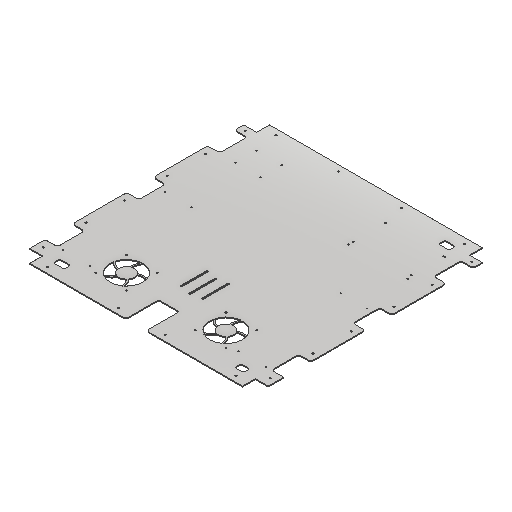
# Autodesk Inventor part: LC_ALU_2mm_Bottom_Plate
Saved by Autodesk Inventor 2026.1 (Build 301233000, 233)
## iProperties
Created: 2016-06-21
Part Number: LC_ALU_2mm_Bottom_Plate
Material: Ogólny
Document SubType Name: Modeling
Designer: Andrzej
Density: 1 g/cm^3
Appearance: Obrobione - aluminium
Mass: 583.865 g
Surface Area: 5900.9 cm^2
Volume: 583.865 cm^3
Author: Andrzej
Autodesk Inventor part; units mm, degrees
ref_plane "YZ Plane" through (0, 0, 0) normal (1, 0, 0) x (0, 1, 0)
ref_plane "XZ Plane" through (0, 0, 0) normal (0, 1, 0) x (-1, 0, 0)
ref_plane "XY Plane" through (0, 0, 0) normal (0, 0, 1) x (1, 0, 0)
sketch "Szkic1" plane through (0, 0, 0) normal (0, 0, 1) x (1, 0, 0)
  line L0 (-788.9548, 119.5598) -> (-788.9548, 95.5598)
  line L1 (-788.9548, 95.5598) -> (-760.4548, 95.5598)
  line L2 (-760.4548, 35.1598) -> (-788.9548, 35.1598)
  line L3 (-788.9548, 35.1598) -> (-788.9548, -94.1902)
  line L4 (-788.9548, -94.1902) -> (-760.4548, -94.1902)
  line L5 (-760.4548, -153.6902) -> (-788.9548, -153.6902)
  line L6 (-788.9548, -153.6902) -> (-788.9548, -283.0402)
  line L7 (-788.9548, -283.0402) -> (-760.4548, -283.0402)
  line L8 (-760.4548, -343.4402) -> (-788.9548, -343.4402)
  line L9 (-788.9548, -343.4402) -> (-788.9548, -382.4402)
  line L10 (-788.9548, -382.4402) -> (-758.9548, -382.4402)
  line L11 (-758.9548, -382.4402) -> (-758.9548, -412.4402)
  line L12 (-758.9548, -412.4402) -> (-259.9548, -412.4402)
  line L13 (-788.9548, 119.5598) -> (-758.9548, 119.5598)
  line L14 (-758.9548, 119.5598) -> (-758.9548, 149.5598)
  line L15 (-758.9548, 149.5598) -> (-259.9548, 149.5598)
  line L16 (-259.9548, -412.4402) -> (-259.9548, -382.4402)
  line L17 (-259.9548, -382.4402) -> (-229.9548, -382.4402)
  line L18 (-259.9548, 149.5598) -> (-259.9548, 119.5598)
  line L19 (-259.9548, 119.5598) -> (-229.9548, 119.5598)
  line L20 (-229.9548, 119.5598) -> (-229.9548, 95.5598)
  line L21 (-229.9548, 95.5598) -> (-258.4548, 95.5598)
  line L22 (-258.4548, 95.5598) -> (-258.4548, 35.1598)
  line L23 (-258.4548, 35.1598) -> (-229.9548, 35.1598)
  line L24 (-229.9548, 35.1598) -> (-229.9548, -94.1902)
  line L25 (-229.9548, -94.1902) -> (-258.4548, -94.1902)
  line L26 (-258.4548, -94.1902) -> (-258.4548, -153.6902)
  line L27 (-258.4548, -153.6902) -> (-229.9548, -153.6902)
  line L28 (-229.9548, -153.6902) -> (-229.9548, -283.0402)
  line L29 (-229.9548, -283.0402) -> (-258.4548, -283.0402)
  line L30 (-258.4548, -343.4402) -> (-229.9548, -343.4402)
  line L31 (-229.9548, -343.4402) -> (-229.9548, -382.4402)
  line L32 (-760.4548, 95.5598) -> (-760.4548, 35.1598)
  line L33 (-760.4548, -283.0402) -> (-760.4548, -343.4402)
  line L34 (-258.4548, -283.0402) -> (-258.4548, -343.4402)
  line L35 (-760.4548, -94.1902) -> (-760.4548, -153.6902)
  line L36 (-261.4548, 148.0598) -> (-757.4548, 148.0598)
  line L37 (-757.4548, 148.0598) -> (-757.4548, 118.0598)
  line L38 (-757.4548, 118.0598) -> (-787.4548, 118.0598)
  line L39 (-787.4548, 118.0598) -> (-787.4548, 97.0598)
  line L40 (-787.4548, 97.0598) -> (-758.9548, 97.0598)
  line L41 (-758.9548, 97.0598) -> (-758.9548, 33.6598)
  line L42 (-758.9548, 33.6598) -> (-787.4548, 33.6598)
  line L43 (-787.4548, 33.6598) -> (-787.4548, -92.6902)
  line L44 (-787.4548, -92.6902) -> (-758.9548, -92.6902)
  line L45 (-758.9548, -92.6902) -> (-758.9548, -155.1902)
  line L46 (-758.9548, -155.1902) -> (-787.4548, -155.1902)
  line L47 (-787.4548, -155.1902) -> (-787.4548, -281.5402)
  line L48 (-787.4548, -281.5402) -> (-758.9548, -281.5402)
  line L49 (-758.9548, -281.5402) -> (-758.9548, -344.9402)
  line L50 (-758.9548, -344.9402) -> (-787.4548, -344.9402)
  line L51 (-787.4548, -344.9402) -> (-787.4548, -380.9402)
  line L52 (-787.4548, -380.9402) -> (-757.4548, -380.9402)
  line L53 (-757.4548, -380.9402) -> (-757.4548, -410.9402)
  line L54 (-757.4548, -410.9402) -> (-261.4548, -410.9402)
  line L55 (-261.4548, -410.9402) -> (-261.4548, -380.9402)
  line L56 (-261.4548, -380.9402) -> (-231.4548, -380.9402)
  line L57 (-231.4548, -380.9402) -> (-231.4548, -344.9402)
  line L58 (-231.4548, -344.9402) -> (-259.9548, -344.9402)
  line L59 (-259.9548, -344.9402) -> (-259.9548, -281.5402)
  line L60 (-259.9548, -281.5402) -> (-231.4548, -281.5402)
  line L61 (-231.4548, -281.5402) -> (-231.4548, -155.1902)
  line L62 (-231.4548, -155.1902) -> (-259.9548, -155.1902)
  line L63 (-259.9548, -155.1902) -> (-259.9548, -92.6902)
  line L64 (-259.9548, -92.6902) -> (-231.4548, -92.6902)
  line L65 (-231.4548, -92.6902) -> (-231.4548, 33.6598)
  line L66 (-231.4548, 33.6598) -> (-259.9548, 33.6598)
  line L67 (-259.9548, 33.6598) -> (-259.9548, 97.0598)
  line L68 (-259.9548, 97.0598) -> (-231.4548, 97.0598)
  line L69 (-231.4548, 97.0598) -> (-231.4548, 118.0598)
  line L70 (-231.4548, 118.0598) -> (-261.4548, 118.0598)
  line L71 (-261.4548, 118.0598) -> (-261.4548, 148.0598)
  line L72 (-533.4548, -410.9402) -> (-533.4548, -334.4402)
  line L73 (-533.4548, -334.4402) -> (-485.4548, -334.4402)
  line L74 (-485.4548, -334.4402) -> (-485.4548, -410.9402)
  line L75 (-534.4548, -280.4402) -> (-534.4548, -220.4402) construction
  line L76 (-532.4548, -280.4402) -> (-532.4548, -220.4402)
  line L77 (-536.4548, -220.4402) -> (-536.4548, -280.4402)
  arc A0 (-536.4548, -280.4402) -> (-532.4548, -280.4402) centre (-534.4548, -280.4402) ccw
  arc A1 (-532.4548, -220.4402) -> (-536.4548, -220.4402) centre (-534.4548, -220.4402) ccw
  line L78 (-509.4548, -285.4402) -> (-509.4548, -225.4402) construction
  line L79 (-507.4548, -285.4402) -> (-507.4548, -225.4402)
  line L80 (-511.4548, -225.4402) -> (-511.4548, -285.4402)
  arc A2 (-511.4548, -285.4402) -> (-507.4548, -285.4402) centre (-509.4548, -285.4402) ccw
  arc A3 (-507.4548, -225.4402) -> (-511.4548, -225.4402) centre (-509.4548, -225.4402) ccw
  line L81 (-484.4548, -280.4402) -> (-484.4548, -220.4402) construction
  line L82 (-482.4548, -280.4402) -> (-482.4548, -220.4402)
  line L83 (-486.4548, -220.4402) -> (-486.4548, -280.4402)
  arc A4 (-486.4548, -280.4402) -> (-482.4548, -280.4402) centre (-484.4548, -280.4402) ccw
  arc A5 (-482.4548, -220.4402) -> (-486.4548, -220.4402) centre (-484.4548, -220.4402) ccw
  line L84 (-726.9548, -382.4402) -> (-709.9548, -382.4402)
  line L85 (-705.9548, -378.4402) -> (-705.9548, -371.4402)
  line L86 (-709.9548, -367.4402) -> (-726.9548, -367.4402)
  line L87 (-730.9548, -371.4402) -> (-730.9548, -378.4402)
  arc A6 (-705.9548, -371.4402) -> (-709.9548, -367.4402) centre (-709.9548, -371.4402) ccw
  arc A7 (-726.9548, -367.4402) -> (-730.9548, -371.4402) centre (-726.9548, -371.4402) ccw
  arc A8 (-730.9548, -378.4402) -> (-726.9548, -382.4402) centre (-726.9548, -378.4402) ccw
  arc A9 (-709.9548, -382.4402) -> (-705.9548, -378.4402) centre (-709.9548, -378.4402) ccw
  line L88 (-315.9548, 104.5598) -> (-298.9548, 104.5598)
  line L89 (-294.9548, 108.5598) -> (-294.9548, 115.5598)
  line L90 (-298.9548, 119.5598) -> (-315.9548, 119.5598)
  line L91 (-319.9548, 115.5598) -> (-319.9548, 108.5598)
  arc A10 (-315.9548, 119.5598) -> (-319.9548, 115.5598) centre (-315.9548, 115.5598) ccw
  arc A11 (-319.9548, 108.5598) -> (-315.9548, 104.5598) centre (-315.9548, 108.5598) ccw
  arc A12 (-298.9548, 104.5598) -> (-294.9548, 108.5598) centre (-298.9548, 108.5598) ccw
  arc A13 (-294.9548, 115.5598) -> (-298.9548, 119.5598) centre (-298.9548, 115.5598) ccw
  line L92 (-665.4548, -357.4402) -> (-585.4548, -357.4402)
  line L93 (-585.4548, -357.4402) -> (-585.4548, -277.4402)
  line L94 (-585.4548, -277.4402) -> (-665.4548, -277.4402)
  line L95 (-665.4548, -277.4402) -> (-665.4548, -357.4402)
  circle A14 centre (-625.4548, -317.4402) radius 38
  line L96 (-752.9548, -352.4402) -> (-675.4548, -352.4402)
  line L97 (-675.4548, -352.4402) -> (-675.4548, -70.9402)
  line L98 (-675.4548, -70.9402) -> (-752.9548, -70.9402)
  line L99 (-752.9548, -70.9402) -> (-752.9548, -352.4402)
  line L100 (-343.4548, -352.4402) -> (-265.9548, -352.4402)
  line L101 (-265.9548, -352.4402) -> (-265.9548, -70.9402)
  line L102 (-265.9548, -70.9402) -> (-343.4548, -70.9402)
  line L103 (-343.4548, -70.9402) -> (-343.4548, -352.4402)
  line L104 (-427.9548, 89.5598) -> (-284.9548, 89.5598)
  line L105 (-427.9548, 89.5598) -> (-427.9548, 5.5598)
  line L106 (-427.9548, 5.5598) -> (-284.9548, 5.5598)
  line L107 (-284.9548, 5.5598) -> (-284.9548, 89.5598)
  line L108 (-427.9548, 5.5598) -> (-427.9548, -5.4402)
  line L109 (-427.9548, -5.4402) -> (-281.4548, -5.4402)
  line L110 (-281.4548, -5.4402) -> (-281.4548, 89.5598)
  line L111 (-281.4548, 89.5598) -> (-284.9548, 89.5598)
  line L112 (-723.9548, 84.5598) -> (-638.9548, 84.5598)
  line L113 (-638.9548, 84.5598) -> (-638.9548, 28.5598)
  line L114 (-638.9548, 28.5598) -> (-723.9548, 28.5598)
  line L115 (-723.9548, 28.5598) -> (-723.9548, 84.5598)
  line L116 (-288.9548, 85.5598) -> (-285.4548, 85.5598) construction
  line L117 (-288.9548, 83.5598) -> (-285.4548, 83.5598)
  line L118 (-285.4548, 87.5598) -> (-288.9548, 87.5598)
  arc A15 (-288.9548, 87.5598) -> (-288.9548, 83.5598) centre (-288.9548, 85.5598) ccw
  arc A16 (-285.4548, 83.5598) -> (-285.4548, 87.5598) centre (-285.4548, 85.5598) ccw
  line L119 (-303.9548, -382.4402) -> (-291.9548, -382.4402)
  line L120 (-287.9548, -378.4402) -> (-287.9548, -371.4402)
  line L121 (-291.9548, -367.4402) -> (-303.9548, -367.4402)
  line L122 (-307.9548, -371.4402) -> (-307.9548, -378.4402)
  arc A17 (-287.9548, -371.4402) -> (-291.9548, -367.4402) centre (-291.9548, -371.4402) ccw
  arc A18 (-303.9548, -367.4402) -> (-307.9548, -371.4402) centre (-303.9548, -371.4402) ccw
  arc A19 (-307.9548, -378.4402) -> (-303.9548, -382.4402) centre (-303.9548, -378.4402) ccw
  arc A20 (-291.9548, -382.4402) -> (-287.9548, -378.4402) centre (-291.9548, -378.4402) ccw
  circle A21 centre (-625.4548, -317.4402) radius 18
  arc A22 (-662.7676, -310.2462) -> (-642.9339, -321.7394) centre (-636.2541, -287.3519) ccw
  arc A23 (-661.9161, -306.7362) -> (-643.4412, -318.141) centre (-635.1638, -284.0659) ccw
  arc A24 (-628.347, -279.5504) -> (-634.0544, -301.6274) centre (-598.7848, -298.9692) ccw
  arc A25 (-624.5951, -279.4499) -> (-630.4705, -300.1532) centre (-595.2035, -298.9764) ccw
  arc A26 (-589.7746, -304.3664) -> (-611.5366, -306.0261) centre (-598.1132, -338.5314) ccw
  arc A27 (-588.6863, -307.8446) -> (-609.4805, -309.1443) centre (-596.9934, -341.9338) ccw
  arc A28 (-601.3141, -346.7869) -> (-610.4589, -327.3963) centre (-635.7941, -351.1964) ccw
  arc A29 (-604.0661, -348.8492) -> (-612.6245, -330.0649) centre (-638.5893, -353.2367) ccw
  arc A30 (-644.1658, -350.5144) -> (-628.3669, -335.2031) centre (-659.1539, -319.2423) ccw
  arc A31 (-647.0681, -348.6951) -> (-631.6229, -334.3504) centre (-661.9, -317.2379) ccw
  line L123 (-433.4548, -357.4402) -> (-353.4548, -357.4402)
  line L124 (-353.4548, -357.4402) -> (-353.4548, -277.4402)
  line L125 (-353.4548, -277.4402) -> (-433.4548, -277.4402)
  line L126 (-433.4548, -277.4402) -> (-433.4548, -357.4402)
  circle A32 centre (-393.4548, -317.4402) radius 38
  circle A33 centre (-393.4548, -317.4402) radius 18
  arc A34 (-430.7676, -310.2462) -> (-410.9339, -321.7394) centre (-404.2541, -287.3519) ccw
  arc A35 (-429.9161, -306.7362) -> (-411.4412, -318.141) centre (-403.1638, -284.0659) ccw
  arc A36 (-396.347, -279.5504) -> (-402.0544, -301.6274) centre (-366.7848, -298.9692) ccw
  arc A37 (-392.5951, -279.4499) -> (-398.4705, -300.1532) centre (-363.2035, -298.9764) ccw
  arc A38 (-357.7746, -304.3664) -> (-379.5366, -306.0261) centre (-366.1132, -338.5314) ccw
  arc A39 (-356.6863, -307.8446) -> (-377.4805, -309.1443) centre (-364.9934, -341.9338) ccw
  arc A40 (-369.3141, -346.7869) -> (-378.4589, -327.3963) centre (-403.7941, -351.1964) ccw
  arc A41 (-372.0661, -348.8492) -> (-380.6245, -330.0649) centre (-406.5893, -353.2367) ccw
  arc A42 (-412.1658, -350.5144) -> (-396.3669, -335.2031) centre (-427.1539, -319.2423) ccw
  arc A43 (-415.0681, -348.6951) -> (-399.6229, -334.3504) centre (-429.9, -317.2379) ccw
  point P0 (0, 0)
  point P1 (-534.4548, -250.4402)
  point P2 (-484.4548, -250.4402)
  point P3 (-509.4548, -255.4402)
  point P4 (-730.9548, -382.4402)
  point P5 (-705.9548, -367.4402)
  point P6 (-705.9548, -382.4402)
  point P7 (-730.9548, -367.4402)
  point P8 (-319.9548, 104.5598)
  point P9 (-294.9548, 119.5598)
  point P10 (-294.9548, 104.5598)
  point P11 (-319.9548, 119.5598)
  point P12 (-661.2048, -353.1902)
  point P13 (-589.7048, -353.1902)
  point P14 (-589.7048, -281.6902)
  point P15 (-661.2048, -281.6902)
  point P16 (-745.9548, -345.4402)
  point P17 (-743.4548, -108.9402)
  point P18 (-682.4548, -345.4402)
  point P19 (-682.4548, -108.9402)
  point P20 (-336.4548, -345.4402)
  point P21 (-333.9548, -108.9402)
  point P22 (-272.9548, -345.4402)
  point P23 (-272.9548, -108.9402)
  point P24 (-369.5, 3)
  point P25 (-423.9548, 85.5598)
  point P26 (-423.9548, 9.5598)
  point P27 (-288.9548, 9.5598)
  point P28 (-423.9548, -1.4402)
  point P29 (-285.4548, -1.4402)
  point P30 (-720.4548, 81.0598)
  point P31 (-720.4548, 32.0598)
  point P32 (-662.4548, 32.0598)
  point P33 (-662.4548, 81.0598)
  point P34 (-287.2048, 85.5598)
  point P35 (-307.9548, -382.4402)
  point P36 (-287.9548, -367.4402)
  point P37 (-287.9548, -382.4402)
  point P38 (-307.9548, -367.4402)
  point P39 (-773.9548, 15.1598)
  point P40 (-773.9548, -74.1902)
  point P41 (-244.9548, 15.1598)
  point P42 (-244.9548, -74.1902)
  point P43 (-244.9548, -173.6902)
  point P44 (-244.9548, -263.0402)
  point P45 (-773.9548, -173.6902)
  point P46 (-773.9548, -263.0402)
  point P47 (-773.9548, -362.9402)
  point P48 (-244.9548, -362.9402)
  point P49 (-728.9548, -397.4402)
  point P50 (-563.4548, -397.4402)
  point P51 (-455.4548, -397.4402)
  point P52 (-289.9548, -397.4402)
  point P53 (-728.9548, 134.5598)
  point P54 (-582.6215, 134.5598)
  point P55 (-436.2881, 134.5598)
  point P56 (-289.9548, 134.5598)
  point P57 (-773.9548, 107.5598)
  point P58 (-244.9548, 107.5598)
  point P59 (-353.4548, -359.2177)
  point P60 (-429.2048, -353.1902)
  point P61 (-357.7048, -353.1902)
  point P62 (-357.7048, -281.6902)
  point P63 (-429.2048, -281.6902)
  dimension "d92" = 76
  dimension "d352" = 36
  dimension "d361" = 76
  dimension "d370" = 36
  dimension "d0" = 30
  dimension "d1" = 30
  dimension "d2" = 30
  dimension "d3" = 30
  dimension "d4" = 30
  dimension "d5" = 30
  dimension "d6" = 30
  dimension "d7" = 30
  dimension "d8" = 559
  dimension "d9" = 562
  dimension "d11" = 559
  dimension "d12" = 60.4
  dimension "d13" = 60.4
  dimension "d14" = 59.5
  dimension "d21" = 54
  dimension "d22" = 69
  dimension "d23" = 243.75
  dimension "d26" = 60.4
  dimension "d27" = 28.5
  dimension "d28" = 28.5
  dimension "d30" = 59.5
  dimension "d31" = 60.4
  dimension "d32" = 69
  dimension "d33" = 243.75
  dimension "d34" = 54
  dimension "d40" = 28.5
  dimension "d42" = 28.5
  dimension "d43" = 28.5
  dimension "d44" = 28.5
  dimension "d45" = 1.5
  dimension "d47" = 76.5
  dimension "d48" = 48
  dimension "d49" = 255.5
  dimension "d50" = 255.5
  dimension "d55" = 405
  dimension "d56" = 25
  dimension "d57" = 25
  dimension "d58" = 5
  dimension "d59" = 5
  dimension "d60" = 502
  dimension "d61" = 251
  dimension "d62" = 30
  dimension "d63" = 4
  dimension "d64" = 30
  dimension "d65" = 4
  dimension "d66" = 30
  dimension "d67" = 4
  dimension "d68" = 25
  dimension "d69" = 15
  dimension "d70" = 28
  dimension "d71" = 30
  dimension "d72" = 4
  dimension "d73" = 4
  dimension "d74" = 4
  dimension "d75" = 4
  dimension "d76" = 30
  dimension "d77" = 25
  dimension "d78" = 15
  dimension "d79" = 35
  dimension "d80" = 4
  dimension "d81" = 4
  dimension "d82" = 4
  dimension "d83" = 4
  dimension "d84" = 80
  constraints: 262 end point, 80 point on circle, 49 perpendicular, 40 centre point, 40 tangent, 35 point on line, 22 parallel, 12 horizontal, 9 vertical, 4 coincident, 4 midpoint, 83 other
  measures "d0" distance between parallel lines of L0 L14
  measures "d1" distance between parallel lines of L15 L13
  measures "d2" distance of L9.end L10.end
  measures "d3" distance of L10.end L11.end
  measures "d4" distance of L12.end L16.end
  measures "d5" distance of L16.end L17.end
  measures "d6" distance of L18.end L19.end
  measures "d7" distance of L15.end L18.end
  measures "d8" distance between parallel lines of L0 L20
  measures "d9" distance between parallel lines of L12 L15
  measures "d11" distance between parallel lines of L31 L9
  measures "d12" distance between parallel lines of L1 L2
  measures "d13" distance between parallel lines of L8 L7
  measures "d14" distance between parallel lines of L4 L5
  measures "d21" distance between parallel lines of L15 L1
  measures "d22" distance between parallel lines of L12 L8
  measures "d23" distance between parallel lines of L15 L4
  measures "d26" distance between parallel lines of L21 L23
  measures "d27" distance of L22.end L23.end
  measures "d28" distance of L24.end L25.end
  measures "d30" distance between parallel lines of L27 L25
  measures "d31" distance between parallel lines of L29 L30
  measures "d32" distance between parallel lines of L12 L30
  measures "d33" distance between parallel lines of L15 L25
  measures "d34" distance between parallel lines of L15 L21
  measures "d40" distance between parallel lines of L0 L32
  measures "d42" distance between parallel lines of L6 L33
  measures "d43" distance between parallel lines of L28 L34
  measures "d44" distance between parallel lines of L3 L35
  measures "d45" distance between parallel lines of L15 L36
  measures "d47" distance of L72.start L72.end
  measures "d48" distance of L72.end L73.end
  measures "d49" distance between parallel lines of L9 L72
  measures "d50" distance between parallel lines of L31 L74
  measures "d55" distance from line of L15 point (-509.455, -255.44)
  measures "d56" horizontal distance of point (-509.455, -255.44) point (-534.455, -250.44)
  measures "d57" horizontal distance of point (-509.455, -255.44) point (-484.455, -250.44)
  measures "d58" vertical distance of point (-534.455, -250.44) point (-509.455, -255.44)
  measures "d59" vertical distance of point (-509.455, -255.44) point (-484.455, -250.44)
  measures "d60" distance between parallel lines of L26 L35
  measures "d61" distance from line of L35 point (-509.455, -255.44)
  measures "d62" distance of point (-534.455, -250.44) L75.end
  measures "d63" diameter of A1
  measures "d64" distance of point (-509.455, -255.44) L78.end
  measures "d65" diameter of A3
  measures "d66" distance of point (-484.455, -250.44) L81.end
  measures "d67" diameter of A5
  measures "d68" distance of point (-730.955, -367.44) point (-705.955, -367.44)
  measures "d69" distance of point (-705.955, -367.44) point (-705.955, -382.44)
  measures "d70" distance between parallel lines of L11 L87
  measures "d71" distance between parallel lines of L84 L12
  measures "d72" radius of A6
  measures "d73" radius of A7
  measures "d74" radius of A8
  measures "d75" radius of A9
  measures "d76" distance between parallel lines of L15 L90
  measures "d77" distance of point (-319.955, 104.56) point (-294.955, 104.56)
  measures "d78" distance of point (-319.955, 119.56) point (-319.955, 104.56)
  measures "d79" distance between parallel lines of L18 L89
  measures "d80" radius of A10
  measures "d81" radius of A11
  measures "d82" radius of A12
  measures "d83" radius of A13
  measures "d84" distance of L94.end L93.end
extrude "Wyciągnięcie proste2" add sketch "Szkic1" along normal blind 2 contours L71 L70 L69 L68 L67 L66 L65 L64 L63 L62 L61 L60 L59 L58 L57 L56 L55 L54 L74 L73 L72 L53 L52 L51 L50 L49 L48 L47 L46 L45 L44 L43 L42 L41 L40 L39 L38 L37 L36 | L54 L72 L73 L74 | A0 L77 A1 L76 | A2 L80 A3 L79 | A4 L83 A5 L82 | A8 L87 A7 L86 A6 L85 A9 L84 | A11 L91 A10 L90 A13 L89 A12 L88 | L95 L94 L93 L92 | A14 A28 A21 A27 | A27 A21 A26 A14 | A14 A29 A21 A28 | A26 A21 A25 A14 | A21 | A14 A30 A21 A29 | A25 A21 A24 A14 | A14 A31 A21 A30 | A24 A21 A23 A14 | A14 A22 A21 A31 | A23 A21 A22 A14 | L99 L98 L97 L96 | L103 L102 L101 L100 | L104 L107 A16 L118 A15 L117 L106 L105 | L111 L110 L109 L108 L106 L107 A16 | A16 L107 | L107 A16 L117 A15 L118 | L112 L113 L114 L115 | A19 L122 A18 L121 A17 L120 A20 L119 | L126 L125 L124 L123 | A32 A40 A33 A39 | A39 A33 A38 A32 | A32 A41 A33 A40 | A38 A33 A37 A32 | A33 | A32 A42 A33 A41 | A37 A33 A36 A32 | A32 A43 A33 A42 | A36 A33 A35 A32 | A32 A34 A33 A43 | A35 A33 A34 A32
fillet "Zaokrąglenie1" radius 6 23 edges at (-758.9548, 97.0598, 1) (-758.9548, 33.6598, 1) (-758.9548, -92.6902, 1) (-758.9548, -155.1902, 1) (-758.9548, -281.5402, 1) (-758.9548, -344.9402, 1) (-259.9548, 97.0598, 1) (-259.9548, 33.6598, 1) (-259.9548, -92.6902, 1) (-259.9548, -155.1902, 1) (-259.9548, -281.5402, 1) (-259.9548, -344.9402, 1) (-787.4548, 97.0598, 1) (-787.4548, 33.6598, 1) (-787.4548, -92.6902, 1) (-787.4548, -155.1902, 1) (-787.4548, -281.5402, 1) (-787.4548, -344.9402, 1) (-231.4548, -281.5402, 1) (-231.4548, -155.1902, 1) (-231.4548, -92.6902, 1) (-231.4548, 33.6598, 1) (-231.4548, 97.0598, 1)
hole "Otwór1" at (-582.6215, 134.5598, 0) at (-436.2881, 134.5598, 0) at (-289.9548, 134.5598, 0) at (-244.9548, 107.5598, 0) at (-244.9548, 15.1598, 0) at (-244.9548, -74.1902, 0) at (-244.9548, -173.6902, 0) at (-244.9548, -263.0402, 0) at (-244.9548, -362.9402, 0) at (-289.9548, -397.4402, 0) at (-455.4548, -397.4402, 0) at (-563.4548, -397.4402, 0) at (-728.9548, -397.4402, 0) at (-773.9548, -362.9402, 0) at (-773.9548, -263.0402, 0) at (-773.9548, -173.6902, 0) at (-773.9548, -74.1902, 0) at (-773.9548, 15.1598, 0) at (-773.9548, 107.5598, 0) at (-728.9548, 134.5598, 0) direction (0, 0, 1) diameter 4 end through all
hole "Otwór4" at (-661.2048, -281.6902, 0) at (-661.2048, -353.1902, 0) at (-589.7048, -281.6902, 0) at (-589.7048, -353.1902, 0) at (-357.7048, -353.1902, 0) at (-357.7048, -281.6902, 0) at (-429.2048, -281.6902, 0) at (-429.2048, -353.1902, 0) direction (0, 0, 1) diameter 4 end through all
hole "Otwór5" at (-682.4548, -345.4402, 0) at (-745.9548, -345.4402, 0) at (-682.4548, -108.9402, 0) at (-743.4548, -108.9402, 0) at (-336.4548, -345.4402, 0) at (-272.9548, -345.4402, 0) at (-272.9548, -108.9402, 0) at (-333.9548, -108.9402, 0) direction (0, 0, 1) diameter 3 end through all
hole "Otwór6" at (-720.4548, 81.0598, 0) at (-720.4548, 32.0598, 0) at (-662.4548, 32.0598, 0) at (-662.4548, 81.0598, 0) direction (0, 0, 1) diameter 3 end through all
hole "Otwór7" at (-423.9548, 85.5598, 0) at (-423.9548, 9.5598, 0) at (-423.9548, -1.4402, 0) at (-288.9548, 9.5598, 0) at (-285.4548, -1.4402, 0) direction (0, 0, 1) diameter 4 end through all
extrude "Wyciągnięcie proste4" cut sketch "Szkic1" along normal blind 10 contours L54 L72 L73 L74 | A0 L77 A1 L76 | A2 L80 A3 L79 | A4 L83 A5 L82 | A8 L87 A7 L86 A6 L85 A9 L84 | A11 L91 A10 L90 A13 L89 A12 L88 | A14 A28 A21 A27 | A26 A21 A25 A14 | A14 A30 A21 A29 | A24 A21 A23 A14 | A14 A22 A21 A31 | A19 L122 A18 L121 A17 L120 A20 L119 | A32 A40 A33 A39 | A38 A33 A37 A32 | A32 A42 A33 A41 | A36 A33 A35 A32 | A32 A34 A33 A43
fillet "Zaokrąglenie5" radius 3 2 edges at (-533.4548, -334.4402, 1) (-485.4548, -334.4402, 1)
fillet "Zaokrąglenie6" radius 6 2 edges at (-533.4548, -410.9402, 1) (-485.4548, -410.9402, 1)
hole "Otwór8" at (-288.9548, 85.5598, 0) at (-285.4548, 85.5598, 0) direction (0, 0, 1) diameter 3 end through all
equation "\"d11\" = d8"
equation "\"d13\" = d12"
equation "\"d26\" = d12"
equation "\"d27\" = d40"
equation "\"d28\" = d40"
equation "\"d30\" = d14"
equation "\"d31\" = d13"
equation "\"d32\" = d22"
equation "\"d33\" = d23"
equation "\"d34\" = d21"
equation "\"d42\" = d40"
equation "\"d43\" = d40"
equation "\"d44\" = d40"
equation "\"d49\" = -0.5 * d48 + 0.5 * d11"
equation "\"d61\" = 0.5 * d60"
equation "\"d64\" = d62"
equation "\"d66\" = d62"
